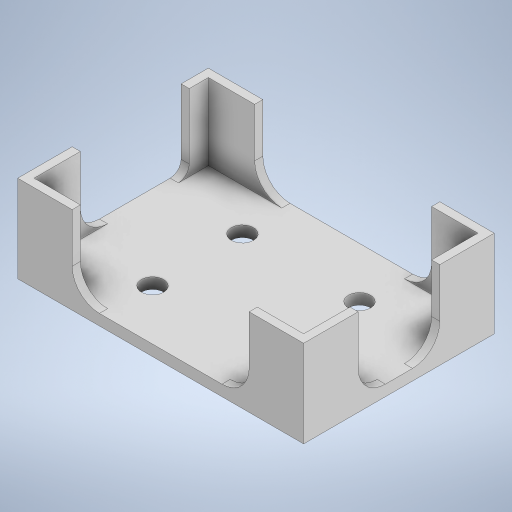
# Autodesk Inventor part: TestingPlatform_base01
Saved by Autodesk Inventor 2024.2 (Build 282272000, 272)
## iProperties
Created: 2024-01-29
Part Number: TestingPlatform_base01
Material: Generic
Document SubType Name: Modeling
Designer: ringl
Density: 1 g/cm^3
Appearance: Default
Author: ringl
Autodesk Inventor part; units mm, degrees
note: some values were not read from the file. Chosen so that the rebuilt part matches the saved one: edges of "Fillet1".
ref_plane "YZ Plane" through (0, 0, 0) normal (1, 0, 0) x (0, 1, 0)
ref_plane "XZ Plane" through (0, 0, 0) normal (0, 1, 0) x (-1, 0, 0)
ref_plane "XY Plane" through (0, 0, 0) normal (0, 0, 1) x (1, 0, 0)
sketch "Sketch1" plane through (0, 0, 0) normal (0, 1, 0) x (-1, 0, 0)
  line L0 (0, 0) -> (58, 0) construction
  line L1 (58, 0) -> (58, -48) construction
  line L2 (58, -48) -> (0, -48) construction
  line L3 (0, -48) -> (0, 0) construction
  circle A0 centre (50.5, -7.5) radius 2.35
  circle A1 centre (50.5, -40.5) radius 2.35
  circle A2 centre (7.5, -7.5) radius 2.35
  circle A3 centre (7.5, -40.5) radius 2.35
  circle A4 centre (50.5, -7.5) radius 5
  circle A5 centre (50.5, -40.5) radius 5
  circle A6 centre (7.5, -7.5) radius 5
  circle A7 centre (7.5, -40.5) radius 5
  dimension "d0" = 58
  dimension "d1" = 48
  dimension "d2" = 4.7
  dimension "d3" = 4.7
  dimension "d4" = 4.7
  dimension "d5" = 4.7
  dimension "d6" = 33
  dimension "d7" = 43
  dimension "d8" = 7.5
  dimension "d9" = 7.5
  dimension "d10" = 7.5
  dimension "d11" = 7.5
  dimension "d12" = 7.5
  dimension "d13" = 7.5
  dimension "d14" = 10
  dimension "d15" = 10
  dimension "d16" = 10
  dimension "d17" = 10
  constraints: 8 centre point, 8 end point, 4 coincident, 2 parallel, 1 horizontal, 1 perpendicular
  measures "d0" distance of L1.end L2.end
  measures "d1" distance of L0.end L1.end
  measures "d2" diameter of A0
  measures "d3" diameter of A1
  measures "d4" diameter of A2
  measures "d5" diameter of A3
  measures "d6" distance of A1.centre A0.centre
  measures "d7" distance of A3.centre A1.centre
  measures "d8" distance from line of L0 A0.centre
  measures "d9" distance from line of L0 A2.centre
  measures "d10" distance from line of L3 A2.centre
  measures "d11" distance from line of L3 A3.centre
  measures "d12" distance from line of L1 A1.centre
  measures "d13" distance from line of L1 A0.centre
  measures "d14" diameter of A4
  measures "d15" diameter of A5
  measures "d16" diameter of A6
  measures "d17" diameter of A7
extrude "Extrusion1" add sketch "Sketch1" along normal blind 12
sketch "Sketch2" plane through (-50.5, 12, -7.5) normal (0, 1, 0) x (1, 0, 0)
  line L0 (-31, -18.5) -> (74, -18.5)
  line L1 (74, -18.5) -> (74, 51.5)
  line L2 (74, 51.5) -> (-31, 51.5)
  line L3 (-31, 51.5) -> (-31, -18.5)
  circle A0 centre (0, 0) radius 2.35 projected
  circle A1 centre (0, 33) radius 2.35 projected
  circle A2 centre (43, 33) radius 2.35 projected
  circle A3 centre (43, 0) radius 2.35 projected
  circle A4 centre (43, 0) radius 2.35
  point P0 (50.5, -7.5)
  dimension "d20" = 105
  dimension "d21" = 70
  dimension "d22" = 18.5
  dimension "d23" = 31
  constraints: 8 end point, 4 coincident, 2 parallel, 1 centre point, 1 horizontal, 1 perpendicular, 1 other
  measures "d20" distance of L2.end L1.end
  measures "d21" distance of L1.end L0.end
  measures "d22" distance from line of L0 point (43, 0)
  measures "d23" distance from line of L3 point (0, 0)
extrude "Extrusion3" add sketch "Sketch2" along normal blind 4
sketch "Sketch3" plane through (-50.5, 16, -7.5) normal (0, 1, 0) x (1, 0, 0)
  line L0 (-31, 51.5) -> (-31, -18.5) projected
  line L1 (-31, -18.5) -> (-31, 1.5)
  line L2 (-31, 1.5) -> (-28, 1.5)
  line L3 (-28, 1.5) -> (-28, -15.5)
  line L4 (-28, -15.5) -> (-11, -15.5)
  line L5 (-11, -15.5) -> (-11, -18.5)
  line L6 (-11, -18.5) -> (-31, -18.5)
  line L7 (-28, 48.5) -> (-11, 48.5)
  line L8 (-11, 48.5) -> (-11, 51.5)
  line L9 (74, -18.5) -> (74, 51.5) projected
  line L10 (74, 51.5) -> (54, 51.5)
  line L11 (54, 51.5) -> (54, 48.5)
  line L12 (71, 31.5) -> (74, 31.5)
  line L13 (74, 31.5) -> (74, 51.5)
  line L14 (74, -18.5) -> (74, 1.5)
  line L15 (74, 1.5) -> (71, 1.5)
  line L16 (71, 1.5) -> (71, -15.5)
  line L17 (71, -15.5) -> (54, -15.5)
  line L18 (54, -15.5) -> (54, -18.5)
  line L19 (54, -18.5) -> (74, -18.5)
  line L20 (74, 51.5) -> (-31, 51.5) projected
  line L21 (54, 48.5) -> (71, 48.5)
  line L22 (71, 48.5) -> (71, 31.5)
  line L23 (-11, 51.5) -> (-31, 51.5)
  line L24 (-31, 51.5) -> (-31, 41.5)
  line L25 (-31, 41.5) -> (-28, 41.5)
  line L26 (-28, 41.5) -> (-28, 48.5)
  point P0 (50.5, -7.5)
  dimension "d28" = 20
  dimension "d37" = 3
  dimension "d48" = 20
  dimension "d49" = 3
  dimension "d50" = 3
  dimension "d51" = 3
  dimension "d52" = 3
  dimension "d53" = 20
  dimension "d54" = 20
  dimension "d55" = 20
  dimension "d56" = 20
  dimension "d57" = 3
  dimension "d58" = 3
  dimension "d69" = 10
  dimension "d70" = 7
  constraints: 48 end point, 15 perpendicular, 8 point on line, 2 collinear, 1 horizontal
  measures "d28" distance of L0.end L1.end
  measures "d37" distance of L10.end L11.end
  measures "d48" distance of L5.end L0.end
  measures "d49" distance of L4.end L5.end
  measures "d50" distance of L1.end L2.end
  measures "d51" distance of L17.end L18.end
  measures "d52" distance of L14.end L15.end
  measures "d53" distance between parallel lines of L19 L15
  measures "d54" distance between parallel lines of L14 L18
  measures "d55" distance of L9.end L10.end
  measures "d56" distance of L12.end L9.end
  measures "d57" distance of L12.start L12.end
  measures "d58" distance of L7.end L8.end
  measures "d69" distance of L0.start L24.end
  measures "d70" distance of L25.end L7.start
extrude "Extrusion4" add sketch "Sketch3" along normal blind 28
fillet "Fillet1" radius 10 7 edges at (-61.5, 16, 9.5) (-80, 16, -9) (-61.5, 16, -57.5) (3.5, 16, -57.5) (22, 16, -39) (22, 16, -9) (3.5, 16, 9.5)
sketch "Sketch4" plane through (-81.5, 12, 11) normal (0, 0, 1) x (1, 0, 0)
  line L0 (0, 0) -> (0, 32) projected
  line L1 (0, 0) -> (100, 0)
  line L2 (100, 0) -> (100, -15)
  line L3 (100, -15) -> (0, -15)
  line L4 (0, -15) -> (0, 0)
  point P0 (81.5, -12)
  dimension "d59" = 100
  dimension "d60" = 15
  constraints: 8 end point, 2 parallel, 1 horizontal, 1 perpendicular
  measures "d59" distance of L2.end L3.end
  measures "d60" distance of L1.end L2.end
extrude "remove legs" cut sketch "Sketch4" against normal through all
sketch "Sketch5" plane through (-50.5, 12, -7.5) normal (0, -1, 0) x (1, 0, 0)
  circle A0 centre (0, 0) radius 2.35 projected
  circle A1 centre (0, 0) radius 4.1
  circle A2 centre (43, 0) radius 2.35 projected
  circle A3 centre (43, 0) radius 4.1
  circle A4 centre (43, -33) radius 2.35 projected
  circle A5 centre (43, -33) radius 4.1
  circle A6 centre (0, -33) radius 2.35 projected
  circle A7 centre (0, -33) radius 4.1
  circle A8 centre (0, 0) radius 2.35
  circle A9 centre (43, 0) radius 2.35
  circle A10 centre (43, -33) radius 2.35
  circle A11 centre (0, -33) radius 2.35
  point P0 (50.5, 7.5)
  dimension "d63" = 8.2
  dimension "d64" = 8.2
  dimension "d65" = 8.2
  dimension "d66" = 8.2
  constraints: 8 centre point, 8 coincident, 4 concentric
  measures "d63" diameter of A1
  measures "d64" diameter of A3
  measures "d65" diameter of A5
  measures "d66" diameter of A7
extrude "Extrusion6" cut sketch "Sketch5" against normal blind 4
fillet "Fillet2" radius 4 1 edges at (-80, 16, -49)
body "Solid1"
